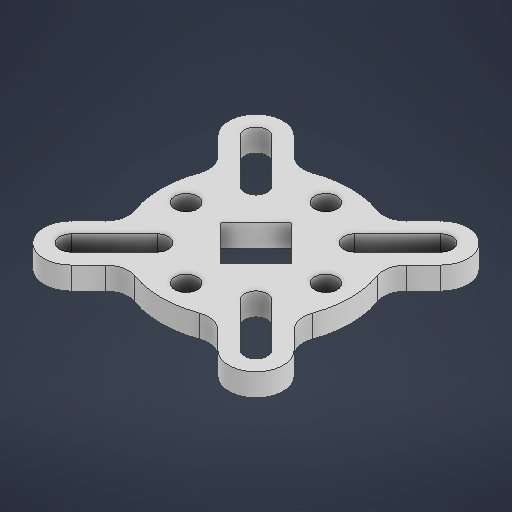
# Autodesk Inventor part: cruceta
Saved by Autodesk Inventor 2026.1 (Build 301233020, 233B)
## iProperties
Created: 2026-02-15
Part Number: cruceta
Material: Generic
Document SubType Name: Modeling
Designer: juanmiguelchungachun
Density: 1 g/cm^3
Appearance: Default
Author: juanmiguelchungachun
Autodesk Inventor part; units mm, degrees
ref_plane "YZ Plane" through (0, 0, 0) normal (1, 0, 0) x (0, 1, 0)
ref_plane "XZ Plane" through (0, 0, 0) normal (0, 1, 0) x (-1, 0, 0)
ref_plane "XY Plane" through (0, 0, 0) normal (0, 0, 1) x (1, 0, 0)
sketch "Sketch1" plane through (0, 0, 0) normal (0, 1, 0) x (-1, 0, 0)
  line L0 (-15.5563, 0) -> (0, -15.5563)
  line L1 (0, -15.5563) -> (15.5563, 0)
  line L2 (15.5563, 0) -> (0, 15.5563)
  line L3 (0, 15.5563) -> (-15.5563, 0)
  line L4 (-15.5563, 0) -> (15.5563, 0) construction
  line L5 (0, -15.5563) -> (0, 15.5563) construction
  circle A0 centre (0, 0) radius 31 construction
  circle A1 centre (31, 0) radius 5
  line L6 (21.9203, -21.9203) -> (41.0122, -41.0122) construction
  line L7 (18.3848, -25.4558) -> (37.4767, -44.5477)
  line L8 (44.5477, -37.4767) -> (25.4558, -18.3848)
  arc A2 (25.4558, -18.3848) -> (18.3848, -25.4558) centre (21.9203, -21.9203) ccw
  arc A3 (37.4767, -44.5477) -> (44.5477, -37.4767) centre (41.0122, -41.0122) ccw
  arc A4 (32.5269, -49.4975) -> (49.4975, -32.5269) centre (41.0122, -41.0122) ccw
  line L9 (49.4975, -32.5269) -> (41.8019, -24.8314)
  line L10 (32.5269, -49.4975) -> (24.8314, -41.8019)
  arc A5 (39.4744, -14.3449) -> (41.8019, -24.8314) centre (48.873, -17.7603) ccw
  arc A6 (24.8314, -41.8019) -> (14.3449, -39.4744) centre (17.7603, -48.873) ccw
  circle A7 centre (0, 31) radius 5
  arc A8 (14.3449, 39.4744) -> (24.8314, 41.8019) centre (17.7603, 48.873) ccw
  line L11 (32.5269, 49.4975) -> (24.8314, 41.8019)
  arc A9 (49.4975, 32.5269) -> (32.5269, 49.4975) centre (41.0122, 41.0122) ccw
  line L12 (49.4975, 32.5269) -> (41.8019, 24.8314)
  arc A10 (41.8019, 24.8314) -> (39.4744, 14.3449) centre (48.873, 17.7603) ccw
  line L13 (25.4558, 18.3848) -> (44.5477, 37.4767)
  line L14 (37.4767, 44.5477) -> (18.3848, 25.4558)
  arc A11 (44.5477, 37.4767) -> (37.4767, 44.5477) centre (41.0122, 41.0122) ccw
  arc A12 (18.3848, 25.4558) -> (25.4558, 18.3848) centre (21.9203, 21.9203) ccw
  circle A13 centre (-31, 0) radius 5
  arc A14 (-39.4744, 14.3449) -> (-41.8019, 24.8314) centre (-48.873, 17.7603) ccw
  line L15 (-49.4975, 32.5269) -> (-41.8019, 24.8314)
  arc A15 (-32.5269, 49.4975) -> (-49.4975, 32.5269) centre (-41.0122, 41.0122) ccw
  line L16 (-32.5269, 49.4975) -> (-24.8314, 41.8019)
  arc A16 (-24.8314, 41.8019) -> (-14.3449, 39.4744) centre (-17.7603, 48.873) ccw
  line L17 (-18.3848, 25.4558) -> (-37.4767, 44.5477)
  line L18 (-44.5477, 37.4767) -> (-25.4558, 18.3848)
  arc A17 (-37.4767, 44.5477) -> (-44.5477, 37.4767) centre (-41.0122, 41.0122) ccw
  arc A18 (-25.4558, 18.3848) -> (-18.3848, 25.4558) centre (-21.9203, 21.9203) ccw
  circle A19 centre (0, -31) radius 5
  arc A20 (-14.3449, -39.4744) -> (-24.8314, -41.8019) centre (-17.7603, -48.873) ccw
  line L19 (-32.5269, -49.4975) -> (-24.8314, -41.8019)
  arc A21 (-49.4975, -32.5269) -> (-32.5269, -49.4975) centre (-41.0122, -41.0122) ccw
  line L20 (-49.4975, -32.5269) -> (-41.8019, -24.8314)
  arc A22 (-41.8019, -24.8314) -> (-39.4744, -14.3449) centre (-48.873, -17.7603) ccw
  line L21 (-25.4558, -18.3848) -> (-44.5477, -37.4767)
  line L22 (-37.4767, -44.5477) -> (-18.3848, -25.4558)
  arc A23 (-44.5477, -37.4767) -> (-37.4767, -44.5477) centre (-41.0122, -41.0122) ccw
  arc A24 (-18.3848, -25.4558) -> (-25.4558, -18.3848) centre (-21.9203, -21.9203) ccw
  arc A25 (-14.3449, -39.4744) -> (14.3449, -39.4744) centre (0, 0) ccw
  arc A26 (-39.4744, 14.3449) -> (-39.4744, -14.3449) centre (0, 0) ccw
  arc A27 (39.4744, -14.3449) -> (39.4744, 14.3449) centre (0, 0) ccw
  arc A28 (14.3449, 39.4744) -> (-14.3449, 39.4744) centre (0, 0) ccw
  point P0 (0, 0)
  point P1 (0, 0)
  point P2 (31.4663, -31.4663)
  dimension "d0" = 22
  dimension "d1" = 62
  dimension "d3" = 5
  dimension "d4" = 45
  dimension "d5" = 45
  dimension "d6" = 58
  dimension "d7" = 5
  dimension "d8" = 12
  dimension "d9" = 10
  dimension "d10" = 10
  dimension "d13" = 360
  dimension "d15" = 42
  constraints: 50 point on circle, 48 end point, 29 centre point, 9 tangent, 7 coincident, 5 midpoint, 5 parallel, 2 perpendicular, 1 horizontal, 1 horizontal alignment, 1 vertical alignment, 105 other
  measures "d0" distance of L0.end L1.end
  measures "d1" diameter of A0
  measures "d3" radius of A1
  measures "d6" distance of L6.end point (0, 0)
  measures "d7" radius of A2
  measures "d8" radius of A4
  measures "d9" radius of A5
  measures "d10" radius of A6
  measures "d15" radius of A25
extrude "Extrusion1" add sketch "Sketch1" along normal blind 10
body "Solid1"
